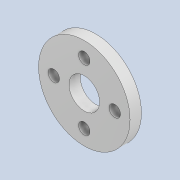
# Autodesk Inventor part: アームモータマウント軸受けパーツ
Saved by Autodesk Inventor 2020.4 (Build 244396000, 396)
## iProperties
Created: 2021-04-23
Part Number: アームモータマウント軸受けパーツ
Material: アルミニウム 2014-T4
Document SubType Name: Modeling
Designer: happy
Density: 2.8 g/cm^3
Appearance: サテン
Author: happy
Autodesk Inventor part; units mm, degrees
ref_plane "YZ Plane" through (0, 0, 0) normal (1, 0, 0) x (0, 1, 0)
ref_plane "XZ Plane" through (0, 0, 0) normal (0, 1, 0) x (-1, 0, 0)
ref_plane "XY Plane" through (0, 0, 0) normal (0, 0, 1) x (1, 0, 0)
sketch "スケッチ1" plane through (0, 0, 0) normal (0, 0, 1) x (1, 0, 0)
  circle A0 centre (96.1098, 17.5902) radius 12.0214
  circle A1 centre (96.1098, 25.6116) radius 1.5
  circle A2 centre (88.0884, 17.5902) radius 1.5
  circle A3 centre (104.1312, 17.5902) radius 1.5
  circle A4 centre (96.1098, 9.5688) radius 1.5
  circle A5 centre (96.1098, 17.5902) radius 4.025
  point P0 (0, 0)
  point P1 (0, 0)
  constraints: 6 centre point, 6 other
extrude "押し出し1" add sketch "スケッチ1" along normal blind 3
